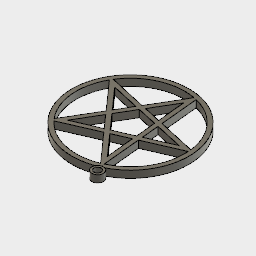
五角星挂件1 (Autodesk Fusion 360 design; units mm, degrees)
Autodesk Fusion 360 part; units mm, degrees
sketch "草图1" plane through (0, 0, 0) normal (0, 1, 0) x (1, 0, 0)
  circle A0 centre (45, -45) radius 40.5649
  line L0 (85.3774, -41.1034) -> (85.4235, -41.1137)
  line L1 (56.619, -34.7234) -> (80.4408, -40.0082)
  arc A1 (82.2844, -40.4172) -> (82.1262, -39.2757) centre (45, -45) ccw
  line L2 (80.4408, -40.0082) -> (82.2844, -40.4172)
  line L3 (56.9209, -37.8633) -> (75.7599, -42.0427)
  line L4 (57.3178, -73.3405) -> (55.4711, -54.1321)
  line L5 (55.1693, -50.9922) -> (51.6928, -14.8318)
  line L6 (75.7599, -42.0427) -> (42.4436, -56.5232)
  line L7 (39.5506, -57.7806) -> (21.853, -65.4727)
  line L8 (31.6494, -48.8472) -> (21.853, -65.4727)
  line L9 (57.3178, -73.3405) -> (33.2508, -46.1296)
  line L10 (31.161, -43.7668) -> (18.3765, -29.3123)
  line L11 (51.6928, -14.8318) -> (41.8964, -31.4572)
  line L12 (40.295, -34.1749) -> (33.2508, -46.1296)
  line L13 (41.8964, -31.4572) -> (53.5395, -34.0402)
  line L14 (37.2155, -33.4917) -> (31.161, -43.7668)
  line L15 (58.0622, -49.7348) -> (54.1032, -8.5547)
  line L16 (53.8, -5.4011) -> (53.7954, -5.354)
  line L17 (53.7954, -5.354) -> (53.7714, -5.3947)
  line L18 (52.163, -8.1243) -> (38.8169, -30.774)
  line L19 (29.5596, -46.4844) -> (12.1427, -26.7923)
  line L20 (10.0437, -24.4192) -> (10.0124, -24.3838)
  line L21 (10.0124, -24.3838) -> (10.0585, -24.394)
  line L22 (13.1515, -25.0802) -> (38.8169, -30.774)
  line L23 (29.5596, -46.4844) -> (16.2134, -69.1341)
  line L24 (14.605, -71.8637) -> (14.581, -71.9045)
  line L25 (41.6404, -60.1434) -> (17.53, -70.6227)
  line L26 (14.6244, -71.8856) -> (14.581, -71.9045)
  line L27 (85.4235, -41.1137) -> (85.3802, -41.1325)
  line L28 (82.4745, -42.3954) -> (44.5334, -58.886)
  line L29 (18.3765, -29.3123) -> (37.2155, -33.4917)
  line L30 (40.295, -34.1749) -> (53.8414, -37.1801)
  arc A2 (82.1262, -39.2757) -> (16.2134, -69.1341) centre (45, -45) ccw
  line L31 (61.1877, -82.2441) -> (61.1563, -82.2087)
  line L32 (59.0574, -79.8355) -> (31.6494, -48.8472)
  line L33 (61.1877, -82.2441) -> (61.1831, -82.197)
  line L34 (60.88, -79.0434) -> (58.3641, -52.8747)
  arc A3 (17.53, -70.6227) -> (59.0574, -79.8355) centre (45, -45) ccw
  arc A4 (60.88, -79.0434) -> (82.4745, -42.3954) centre (45, -45) ccw
  point P0 (45, -45)
extrude "拉伸1" add sketch "草图1" along normal blind 5 contours A0 makes body 1
sketch "草图2" plane through (0, 0, 0) normal (0, 1, 0) x (1, 0, 0)
  circle A0 centre (-40, -40) radius 2.5
  circle A1 centre (-40, -40) radius 4
extrude "拉伸2" add sketch "草图2" along normal blind 5 separate body makes body 2
move_body "移动1" bodies 2 to x (1, 0, 0) y (0, 1, 0) z (0, 0, 1) at (100, 0, 40)
move_body "移动2" bodies 2 to x (1, 0, 0) y (0, 1, 0) z (0, 0, 1) at (2.5602, 0, 4.7305)
move_body "移动3" bodies 2 to x (1, 0, 0) y (0, 1, 0) z (0, 0, 1) at (-0.319, 0.0117, 0.2823)
combine "合并1" operation add target body 1 tool bodies 2
